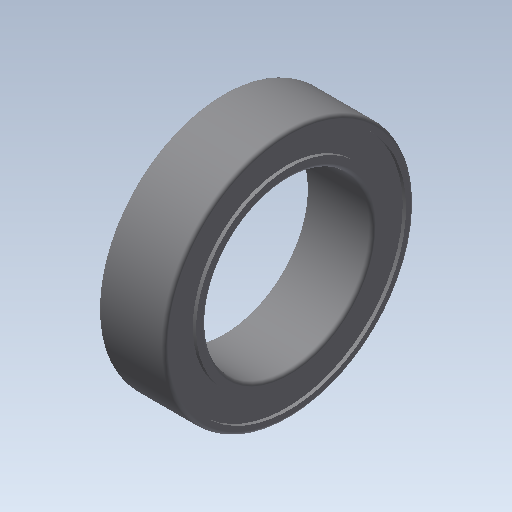
# Autodesk Inventor part: B6700ZZ
Saved by Autodesk Inventor 2020 (Build 240168000, 168)
## iProperties
Created: 2018-12-11
Part Number: B6700ZZ
Material: Generic
Catalog Web Link: www.cadenas.de
Description: B6_ _ _ZZ, SB6_ _ _ZZ-Deep Groove Ball Bearings - Double Shield Type
Vendor: MISUMI
Document SubType Name: Modeling
Designer: psadmin
Manufacturer: MISUMI
Mass: 0.368831 g
Surface Area: 5.28742 cm^2
Volume: 0.368831 cm^3
Density: 1 g/cm^3
Appearance: PSOLRGB-175-175-175
Category: PARTsolutions
Company: MISUMI
PSOL_IDENT_0: {$CADENAS_DATA\23d-libs\misumi\metric\12_bearing_holders\sb6010zz.prj},171 {VTYP=3D},{NB=B6700ZZ},{L
PSOL_IDENT_1: INA=B6700ZZ},{NN=B6_ _ _ZZ, SB6_ _ _ZZ},{DATE=30.03.2018 01:49:31},{GEOMDATE=29.07.2009 00:00:00},{V
PSOL_IDENT_2: ERSION=},{LINEID=10},{WBVAR=TS},{WBNUMERIC=}  {NB=B6700ZZ},{LINA=B6700ZZ},{KT=DUMMY},{PN=B6700ZZ},{T
PSOL_IDENT_3: S=},{TS1= '', 'Steel', 'S', 'Stainless Steel'},{MAT=52100 Bearing Steel},{BN=6700ZZ},{DD=10},{D=15},
PSOL_IDENT_4: {B=4},{RR=0.2},{CR=0.85},{COR=0.43},{CRS=0.85},{CRSS=0.68},{CORS=0.43},{CORSS=0.34},{DD1=1.000},{R1=
PSOL_IDENT_5: 1.000},{R2=1.000},{DSMIN=10.4},{DSMAX=11.21},{DS1=11.21},{DDHH=14.2},{R=0.2},{MASS=2},{MASS11=2},{AA=
PSOL_IDENT_6: 3.6000},{BB=0.4800},{CC=0.6000},{TYS=w/o Retaining Ring}
NN: B6_ _ _ZZ, SB6_ _ _ZZ
NT: Deep Groove Ball Bearings - Double Shield Type
NB: B6700ZZ
NBSYN: $PN.
LINA: B6700ZZ
PN: B6700ZZ
TS: Steel
MAT: 52100 Bearing Steel
BN: 6700ZZ
DD: 10
D: 15
B: 4
RR: 0.2
CR: 0.85
COR: 0.43
DSMIN: 10.4
DSMAX: 11.21
DDHH: 14.2
R: 0.2
MASS: 2
SUPPLIER: MISUMI
ARTICLENO: B6700ZZ
BOMINFO: B6700ZZ
CREATOR: CADENAS GmbH
Title: B6700ZZ
Author: Cadenas PARTsolutions
Comments: Deep Groove Ball Bearings - Double Shield Type
Autodesk Inventor part; units mm, degrees
sketch "Sketch_1" plane through (0, 0, 0) normal (0, 0, 1) x (1, 0, 0)
  line L0 (4, 0) -> (0, 0)
  arc A0 (0, 5.2) -> (0.2, 5) centre (0.2, 5.2) ccw
  line L1 (0.2, 5) -> (3.8, 5)
  arc A1 (3.8, 5) -> (4, 5.2) centre (3.8, 5.2) ccw
  line L2 (4, 5.2) -> (4, 5.6)
  line L3 (4, 5.6) -> (3.8, 5.6)
  line L4 (3.8, 5.6) -> (3.8, 7.02)
  line L5 (3.8, 7.02) -> (4, 7.02)
  line L6 (4, 7.02) -> (4, 7.3)
  arc A2 (4, 7.3) -> (3.8, 7.5) centre (3.8, 7.3) ccw
  line L7 (3.8, 7.5) -> (0.2, 7.5)
  arc A3 (0.2, 7.5) -> (0, 7.3) centre (0.2, 7.3) ccw
  line L8 (0, 7.3) -> (0, 7.02)
  line L9 (0, 7.02) -> (0.2, 7.02)
  line L10 (0.2, 7.02) -> (0.2, 5.6)
  line L11 (0.2, 5.6) -> (0, 5.6)
  line L12 (0, 5.6) -> (0, 5.2)
  constraints: 26 end point, 8 point on circle, 4 centre point
revolve "Revolution1" add sketch "Sketch_1" angle 360 about axis through (4, 0, 0) along (1, 0, 0)
ref_plane "center_point_XY" through (2, 0, 0) normal (1, 0, 0) x (0, 0, -1)
ref_plane "center_point_YZ" through (2, 0, 0) normal (0, 0, -1) x (0, 1, 0)
ref_plane "center_point_ZX" through (2, 0, 0) normal (0, 1, 0) x (1, 0, 0)
ref_plane "to_housing_XY" through (0, 0, 0) normal (1, 0, 0) x (0, 0, -1)
ref_plane "to_housing_YZ" through (0, 0, 0) normal (0, 0, -1) x (0, 1, 0)
ref_plane "to_housing_ZX" through (0, 0, 0) normal (0, 1, 0) x (1, 0, 0)
ref_plane "to_ring_XY" through (3.6, 0, 0) normal (1, 0, 0) x (0, 0, -1)
ref_plane "to_ring_YZ" through (3.6, 0, 0) normal (0, 0, -1) x (0, 1, 0)
ref_plane "to_ring_ZX" through (3.6, 0, 0) normal (0, 1, 0) x (1, 0, 0)
body "Solid1"
